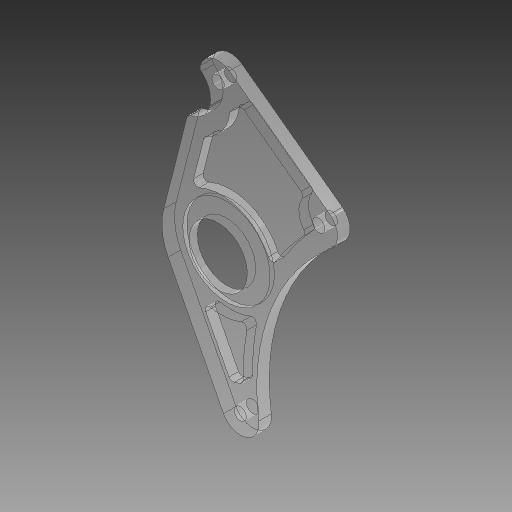
# Autodesk Inventor part: 前脚軸抑え1
Saved by Autodesk Inventor 2020 (Build 240168000, 168)
## iProperties
Created: 2019-09-03
Part Number: 前脚軸抑え1
Material: ポリカーボネート、クリア
Document SubType Name: Modeling
Designer: 雪村
Density: 1.2 g/cm^3
Appearance: ポリカーボネート - クリア
Mass: 3.69667 g
Surface Area: 40.5739 cm^2
Volume: 3.08056 cm^3
Description: ポリカ 3t
Author: 雪村
Autodesk Inventor part; units mm, degrees
ref_plane "YZ Plane" through (0, 0, 0) normal (1, 0, 0) x (0, 1, 0)
ref_plane "XZ Plane" through (0, 0, 0) normal (0, 1, 0) x (-1, 0, 0)
ref_plane "XY Plane" through (0, 0, 0) normal (0, 0, 1) x (1, 0, 0)
sketch "スケッチ1" plane through (0, 0, 0) normal (0, 0, 1) x (1, 0, 0)
  circle A0 centre (117.7963, 39.9634) radius 1.5
  circle A1 centre (136.6898, 88.5769) radius 1.5
  circle A2 centre (112.5, 106.321) radius 1.5
  circle A3 centre (112.5, 70) radius 7.025
  circle A4 centre (112.5, 106.321) radius 4.5
  circle A5 centre (136.6898, 88.5769) radius 4.5
  circle A6 centre (117.7963, 39.9634) radius 4.5
  circle A7 centre (112.5, 70) radius 13.5
  line L0 (113.7925, 37.909) -> (100.4888, 63.837)
  line L1 (99.421, 73.3452) -> (108.1403, 107.436)
  line L2 (115.1616, 109.9495) -> (139.3514, 92.2054)
  arc A8 (139.5498, 85.1026) -> (122.2518, 40.5945) centre (170.5554, 47.4369) ccw
  circle A9 centre (112.5, 70) radius 10.5 construction
  point P0 (0, 0)
  point P1 (0, 0)
  dimension "d0" = 9
  dimension "d1" = 9
  dimension "d2" = 9
  dimension "d6" = 3
  dimension "d7" = 3
  dimension "d8" = 3
  dimension "d28" = 21
  dimension "d29" = 3
  constraints: 10 centre point, 10 point on circle, 9 tangent, 6 end point, 4 coincident, 4 other
  measures "d0" diameter of A4
  measures "d1" diameter of A5
  measures "d2" diameter of A6
  measures "d6" diameter of A2
  measures "d7" diameter of A1
  measures "d8" diameter of A0
  measures "d28" diameter of A9
  measures "d29" radial gap between concentric circles of A7 A9
extrude "押し出し1" add sketch "スケッチ1" along normal blind 3
shell "シェル1" thickness 4 removed faces 2 at (121.0855, 90.1409, 0) at (121.0855, 90.1409, 3)
fillet "フィレット1" radius 1 10 edges at (119.7254, 61.6727, 1.5) (117.8065, 45.4634, 1.5) (106.6018, 60.6854, 1.5) (114.851, 44.6083, 1.5) (123.4525, 71.2625, 1.5) (104.6826, 77.7742, 1.5) (132.9833, 84.5135, 1.5) (132.5691, 92.2197, 1.5) (117.2122, 103.4845, 1.5) (110.6584, 101.1385, 1.5)
sketch "スケッチ2" plane through (0, 0, 3) normal (0, 0, 1) x (1, 0, 0)
  line L0 (105.404, 80.5947) -> (110.4097, 100.1662) projected
  arc A0 (111.5511, 100.9035) -> (110.4097, 100.1662) centre (111.3785, 99.9184) ccw projected
  arc A1 (111.5511, 100.9035) -> (116.6714, 102.7364) centre (112.5, 106.321) ccw projected
  arc A2 (118.0213, 102.891) -> (116.6714, 102.7364) centre (117.4299, 102.0847) ccw projected
  line L1 (118.0213, 102.891) -> (131.76, 92.8132) projected
  arc A3 (132.0179, 91.4792) -> (131.76, 92.8132) centre (131.1685, 92.0069) ccw projected
  arc A4 (132.0179, 91.4792) -> (132.3871, 85.1511) centre (136.6898, 88.5769) ccw projected
  arc A5 (132.329, 83.8386) -> (132.3871, 85.1511) centre (131.6048, 84.5282) ccw projected
  arc A6 (132.329, 83.8386) -> (124.6885, 73.563) centre (170.5554, 47.4369) ccw projected
  arc A7 (122.8783, 73.7205) -> (124.6885, 73.563) centre (123.8196, 74.0579) ccw projected
  arc A8 (122.8783, 73.7205) -> (106.8823, 79.4864) centre (112.5, 70) ccw projected
  arc A9 (105.404, 80.5947) -> (106.8823, 79.4864) centre (106.3728, 80.3469) ccw projected
  line L2 (114.3929, 45.5011) -> (107.9308, 58.0953) projected
  arc A10 (109.1265, 59.5038) -> (107.9308, 58.0953) centre (108.8205, 58.5518) ccw projected
  arc A11 (109.1265, 59.5038) -> (117.642, 60.2476) centre (112.5, 70) ccw projected
  arc A12 (119.0836, 59.1413) -> (117.642, 60.2476) centre (118.1084, 59.363) ccw projected
  arc A13 (119.0836, 59.1413) -> (117.7797, 46.403) centre (170.5554, 47.4369) ccw projected
  arc A14 (116.9363, 45.3957) -> (117.7797, 46.403) centre (116.7799, 46.3834) ccw projected
  arc A15 (116.9363, 45.3957) -> (115.6693, 45.0354) centre (117.7963, 39.9634) ccw projected
  arc A16 (114.3929, 45.5011) -> (115.6693, 45.0354) centre (115.2826, 45.9576) ccw projected
  arc A17 (139.5498, 85.1026) -> (122.2518, 40.5945) centre (170.5554, 47.4369) ccw projected
  arc A18 (139.5498, 85.1026) -> (139.3514, 92.2054) centre (136.6898, 88.5769) ccw projected
  line L3 (139.3514, 92.2054) -> (115.1616, 109.9495) projected
  arc A19 (115.1616, 109.9495) -> (108.1403, 107.436) centre (112.5, 106.321) ccw projected
  line L4 (108.1403, 107.436) -> (99.421, 73.3452) projected
  arc A20 (99.421, 73.3452) -> (100.4888, 63.837) centre (112.5, 70) ccw projected
  line L5 (100.4888, 63.837) -> (113.7925, 37.909) projected
  arc A21 (113.7925, 37.909) -> (122.2518, 40.5945) centre (117.7963, 39.9634) ccw projected
  circle A22 centre (136.6898, 88.5769) radius 1.5 projected
  circle A23 centre (112.5, 106.321) radius 1.5 projected
  circle A24 centre (112.5, 70) radius 7.025 projected
  circle A25 centre (117.7963, 39.9634) radius 1.5 projected
  point P0 (0, 0)
extrude "押し出し2" add sketch "スケッチ2" against normal blind 0.7 contours L0 A0 A1 A2 L1 A3 A4 A5 A6 A7 A8 A9 | L2 A10 A11 A12 A13 A14 A15 A16
sketch "スケッチ4" plane through (0, 0, 3) normal (0, 0, 1) x (1, 0, 0)
  arc A0 (139.5498, 85.1026) -> (122.2518, 40.5945) centre (170.5554, 47.4369) ccw projected
  arc A1 (139.5498, 85.1026) -> (139.3514, 92.2054) centre (136.6898, 88.5769) ccw projected
  line L0 (139.3514, 92.2054) -> (115.1616, 109.9495) projected
  arc A2 (115.1616, 109.9495) -> (108.1403, 107.436) centre (112.5, 106.321) ccw projected
  line L1 (108.1403, 107.436) -> (99.421, 73.3452) projected
  arc A3 (99.421, 73.3452) -> (100.4888, 63.837) centre (112.5, 70) ccw projected
  line L2 (100.4888, 63.837) -> (113.7925, 37.909) projected
  arc A4 (113.7925, 37.909) -> (122.2518, 40.5945) centre (117.7963, 39.9634) ccw projected
  circle A5 centre (136.6898, 88.5769) radius 1.5 projected
  circle A6 centre (112.5, 106.321) radius 1.5 projected
  circle A7 centre (112.5, 70) radius 7.025 projected
  circle A8 centre (117.7963, 39.9634) radius 1.5 projected
  circle A9 centre (112.5, 106.321) radius 3
  circle A10 centre (104.6846, 101.8578) radius 6
  line L3 (104.6846, 101.8578) -> (136.6898, 88.5769)
  point P0 (0, 0)
  dimension "d16" = 6
  dimension "d17" = 12
  dimension "d18" = 34.6513
  constraints: 2 centre point, 2 end point, 1 coincident, 1 tangent
  measures "d16" diameter of A9
  measures "d17" diameter of A10
  measures "d18" distance of L3.start L3.end
extrude "押し出し3" cut sketch "スケッチ4" against normal through all contours A10 L3 L1 | L1 A10 | L1 L3 A10
sketch "スケッチ5" plane through (0, 0, 0) normal (0, 0, -1) x (-1, 0, 0)
  arc A0 (-107.9937, 106.8628) -> (-105.1843, 95.8786) centre (-104.6846, 101.8578) ccw projected
  arc A1 (-110.2456, 110.169) -> (-106.949, 92.1175) centre (-104.6846, 101.8578) ccw
  arc A2 (-116.6714, 102.7364) -> (-111.5511, 100.9035) centre (-112.5, 106.321) ccw projected
  arc A3 (-110.4097, 100.1662) -> (-111.5511, 100.9035) centre (-111.3785, 99.9184) ccw projected
  line L0 (-110.4097, 100.1662) -> (-105.404, 80.5947) projected
  point P0 (0, 0)
  point P1 (-114.6671, 101.2659)
  point P2 (-108.4756, 92.6042)
  dimension "d21" = 4
  constraints: 2 point on circle, 1 centre point
  measures "d21" radial gap between concentric circles of A0 A1
extrude "押し出し4" add sketch "スケッチ5" against normal blind 3
fillet "フィレット2" radius 1 4 edges at (107.9937, 106.8628, 1.5) (105.1843, 95.8786, 1.5) (108.4756, 92.6042, 1.15) (114.6671, 101.2659, 1.15)
sketch "スケッチ6" plane through (0, 0, 0) normal (0, 0, -1) x (-1, 0, 0)
  circle A0 centre (-112.5, 70) radius 7.025 projected
  circle A1 centre (-112.5, 70) radius 10.5
  point P0 (0, 0)
  dimension "d25" = 21
  constraints: 1 centre point, 1 coincident
  measures "d25" diameter of A1
extrude "押し出し5" cut sketch "スケッチ6" against normal blind 1
sketch "スケッチ7" plane through (0, 0, 0) normal (0, 0, -1) x (-1, 0, 0)
  arc A0 (-106.8823, 79.4864) -> (-122.8783, 73.7205) centre (-112.5, 70) ccw projected
  arc A1 (-117.642, 60.2476) -> (-119.0836, 59.1413) centre (-118.1084, 59.363) ccw projected
  arc A2 (-117.642, 60.2476) -> (-109.1265, 59.5038) centre (-112.5, 70) ccw projected
  arc A3 (-107.9308, 58.0953) -> (-109.1265, 59.5038) centre (-108.8205, 58.5518) ccw projected
  circle A4 centre (-112.5, 70) radius 10.5 projected
  circle A5 centre (-112.5, 70) radius 12.5
  arc A6 (-124.6885, 73.563) -> (-122.8783, 73.7205) centre (-123.8196, 74.0579) ccw projected
  arc A7 (-106.8823, 79.4864) -> (-105.404, 80.5947) centre (-106.3728, 80.3469) ccw projected
  line L0 (-108.3547, 92.1316) -> (-105.404, 80.5947) projected
  point P0 (0, 0)
  point P1 (-119.1081, 59.3895)
  point P2 (-107.8314, 58.4046)
  point P3 (-105.3757, 80.271)
  point P4 (-124.539, 73.3633)
  dimension "d30" = 2
  constraints: 1 centre point
  measures "d30" radial gap between concentric circles of A4 A5
extrude "押し出し6" add sketch "スケッチ7" against normal blind 3 contours A0 A6 A5 A7 | A1 A2 A3 A5
fillet "フィレット3" radius 1 4 edges at (124.539, 73.3633, 1.15) (105.3757, 80.271, 1.15) (107.8314, 58.4046, 1.15) (119.1081, 59.3895, 1.15)
sketch "スケッチ8" plane through (0, 0, 0) normal (0, 0, -1) x (-1, 0, 0)
  circle A0 centre (-112.5, 70) radius 10.5 projected
  arc A1 (-107.2814, 81.3585) -> (-105.8951, 82.515) centre (-106.8639, 82.2672) ccw projected
  arc A2 (-107.2814, 81.3585) -> (-123.8535, 75.2295) centre (-112.5, 70) ccw projected
  arc A3 (-125.6132, 75.1234) -> (-123.8535, 75.2295) centre (-124.7618, 75.6479) ccw projected
  arc A4 (-125.6132, 75.1234) -> (-132.329, 83.8386) centre (-170.5554, 47.4369) ccw projected
  arc A5 (-132.3871, 85.1511) -> (-132.329, 83.8386) centre (-131.6048, 84.5282) ccw projected
  arc A6 (-132.3871, 85.1511) -> (-132.0179, 91.4792) centre (-136.6898, 88.5769) ccw projected
  arc A7 (-131.76, 92.8132) -> (-132.0179, 91.4792) centre (-131.1685, 92.0069) ccw projected
  line L0 (-131.76, 92.8132) -> (-118.0213, 102.891) projected
  arc A8 (-116.6714, 102.7364) -> (-118.0213, 102.891) centre (-117.4299, 102.0847) ccw projected
  arc A9 (-116.6714, 102.7364) -> (-115.1351, 101.4933) centre (-112.5, 106.321) ccw projected
  arc A10 (-114.6207, 100.7285) -> (-115.1351, 101.4933) centre (-115.6143, 100.6156) ccw projected
  arc A11 (-114.6207, 100.7285) -> (-108.9018, 92.7905) centre (-104.6846, 101.8578) ccw projected
  arc A12 (-108.3547, 92.1316) -> (-108.9018, 92.7905) centre (-109.3235, 91.8838) ccw projected
  line L1 (-108.3547, 92.1316) -> (-105.8951, 82.515) projected
  arc A13 (-105.0179, 95.2278) -> (-105.8007, 95.9625) centre (-105.9867, 94.98) ccw projected
  arc A14 (-110.3056, 99.759) -> (-105.8007, 95.9625) centre (-104.6846, 101.8578) ccw projected
  line L2 (-110.3056, 99.759) -> (-110.4097, 100.1662) projected
  arc A15 (-110.4097, 100.1662) -> (-110.507, 100.4089) centre (-111.3785, 99.9184) ccw projected
  arc A16 (-108.4948, 106.4928) -> (-110.507, 100.4089) centre (-104.6846, 101.8578) ccw projected
  arc A17 (-108.4948, 106.4928) -> (-108.1669, 107.535) centre (-109.1298, 107.2653) ccw projected
  arc A18 (-108.1669, 107.535) -> (-115.1616, 109.9495) centre (-112.5, 106.321) ccw projected
  line L3 (-139.3514, 92.2054) -> (-115.1616, 109.9495) projected
  arc A19 (-139.3514, 92.2054) -> (-139.5498, 85.1026) centre (-136.6898, 88.5769) ccw projected
  arc A20 (-122.2518, 40.5945) -> (-139.5498, 85.1026) centre (-170.5554, 47.4369) ccw projected
  arc A21 (-122.2518, 40.5945) -> (-113.7925, 37.909) centre (-117.7963, 39.9634) ccw projected
  line L4 (-100.4888, 63.837) -> (-113.7925, 37.909) projected
  arc A22 (-100.4888, 63.837) -> (-99.421, 73.3452) centre (-112.5, 70) ccw projected
  line L5 (-105.0179, 95.2278) -> (-99.421, 73.3452) projected
  arc A23 (-117.3423, 58.476) -> (-118.7118, 57.366) centre (-117.7297, 57.5541) ccw projected
  arc A24 (-117.3423, 58.476) -> (-109.9309, 57.7669) centre (-112.5, 70) ccw projected
  arc A25 (-108.8357, 56.3317) -> (-109.9309, 57.7669) centre (-109.7254, 56.7882) ccw projected
  line L6 (-108.8357, 56.3317) -> (-114.3929, 45.5011) projected
  arc A26 (-115.6693, 45.0354) -> (-114.3929, 45.5011) centre (-115.2826, 45.9576) ccw projected
  arc A27 (-115.6693, 45.0354) -> (-116.9363, 45.3957) centre (-117.7963, 39.9634) ccw projected
  arc A28 (-117.7797, 46.403) -> (-116.9363, 45.3957) centre (-116.7799, 46.3834) ccw projected
  arc A29 (-117.7797, 46.403) -> (-118.7118, 57.366) centre (-170.5554, 47.4369) ccw projected
  circle A30 centre (-136.6898, 88.5769) radius 1.5 projected
  circle A31 centre (-112.5, 106.321) radius 1.5 projected
  circle A32 centre (-117.7963, 39.9634) radius 1.5 projected
  circle A33 centre (-112.5, 70) radius 7.025 projected
  point P0 (0, 0)
